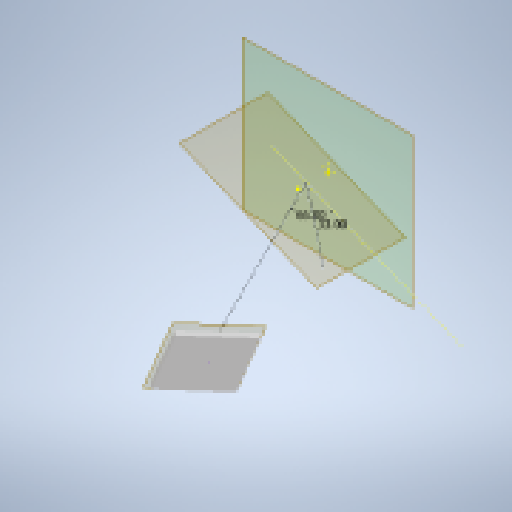
# Autodesk Inventor part: Część10
Saved by Autodesk Inventor 2025.1 (Build 291241020, 241B)
## iProperties
Created: 2024-10-13
Part Number: Część10
Material: Ogólny
Document SubType Name: Modeling
Designer: zychlix
Density: 1 g/cm^3
Appearance: Domyślna
Author: zychlix
Autodesk Inventor part; units mm, degrees
ref_plane "YZ Plane" through (0, 0, 0) normal (1, 0, 0) x (0, 1, 0)
ref_plane "XZ Plane" through (0, 0, 0) normal (0, 1, 0) x (-1, 0, 0)
ref_plane "XY Plane" through (0, 0, 0) normal (0, 0, 1) x (1, 0, 0)
ref_plane "Płaszczyzna konstrukcyjna2" through (-0.19, 0, -10) normal (0, 0, -1) x (-1, 0, 0)
sketch "Szkic1" plane through (-0.19, 0, -10) normal (0, 0, -1) x (-1, 0, 0)
  point P0 (-0.19, 0)
  point P1 (-0.19, 0.975)
ref_plane "Płaszczyzna konstrukcyjna3" through (0, 0.975, -3) normal (0.3826834, 0.9238795, 0) x (0.9238795, -0.3826834, 0)
sketch "Szkic2" plane through (0, 0.975, -3) normal (0.3826834, 0.9238795, 0) x (0.9238795, -0.3826834, 0)
  line L0 (0, 0) -> (20.3949, -13.2446) construction
  line L1 (0, 0) -> (24.6472, -55.3585) construction
  line L2 (53.7615, 0) -> (-12.2572, 0) construction
  point P0 (0.3731, -3)
  point P1 (24.3225, -54.6292)
  dimension "d0" = 33
  dimension "d1" = 66
  constraints: 4 end point, 1 point on line
  measures "d0" angle of L0 L2
  measures "d1" angle of L1 L2
ref_plane "Płaszczyzna konstrukcyjna4" through (22.471, -8.3328, 51.6292) normal (0.7748306, -0.3209453, 0.544639) x (0.3826834, 0.9238795, 0)
sketch "Szkic3" plane through (22.471, -8.3328, 51.6292) normal (0.7748306, -0.3209453, 0.544639) x (0.3826834, 0.9238795, 0)
  line L0 (-10.4423, 9.7716) -> (9.5577, 9.7716)
  line L1 (9.5577, 9.7716) -> (9.5577, -10.2284)
  line L2 (9.5577, -10.2284) -> (-10.4423, -10.2284)
  line L3 (-10.4423, -10.2284) -> (-10.4423, 9.7716)
  point P0 (-0.9008, -30.2561)
  dimension "d2" = 20
  dimension "d3" = 20
  constraints: 8 end point, 2 parallel, 1 horizontal, 1 perpendicular
  measures "d2" distance of L0.start L0.end
  measures "d3" distance of L0.end L1.end
extrude "Wyciągnięcie proste1" add sketch "Szkic3" along normal blind 1.5
